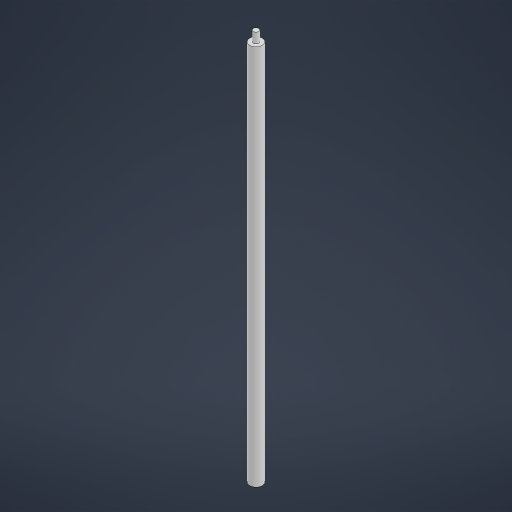
# Autodesk Inventor part: BaseSpacer_M3
Saved by Autodesk Inventor 2024.2 (Build 282272000, 272)
## iProperties
Created: 2023-12-28
Part Number: BaseSpacer_M3
Material: 一般
Document SubType Name: Modeling
Designer: Hanaoka
Density: 1 g/cm^3
Appearance: 既定
Author: Hanaoka
Autodesk Inventor part; units mm, degrees
ref_plane "YZ Plane" through (0, 0, 0) normal (1, 0, 0) x (0, 1, 0)
ref_plane "XZ Plane" through (0, 0, 0) normal (0, 1, 0) x (-1, 0, 0)
ref_plane "XY Plane" through (0, 0, 0) normal (0, 0, 1) x (1, 0, 0)
sketch "スケッチ2" plane through (0, 0, 0) normal (0, 0, 1) x (1, 0, 0)
  line L0 (0, 0) -> (2.5, 0)
  line L1 (2.5, 0) -> (2.5, 150)
  line L2 (2.5, 150) -> (0, 150)
  line L3 (0, 150) -> (0, 0)
  line L4 (1.1, 0) -> (1.1, 6)
  line L5 (1.1, 6) -> (0, 6)
  line L6 (1.1, 150) -> (1.1, 154)
  line L7 (1.1, 154) -> (0, 154)
  line L8 (0, 154) -> (0, 150)
  dimension "d4" = 2.5
  dimension "d5" = 150
  dimension "d6" = 1.1
  dimension "d7" = 6
  dimension "d8" = 1.1
  dimension "d9" = 4
  constraints: 18 end point, 5 perpendicular, 4 point on line, 3 vertical, 1 horizontal
  measures "d4" distance of L0.start L0.end
  measures "d5" distance of L0.end L1.end
  measures "d6" distance of L4.end L5.end
  measures "d7" distance of L4.start L4.end
  measures "d8" distance of L6.end L7.end
  measures "d9" distance of L6.start L6.end
revolve "回転1" add sketch "スケッチ2" angle 360 about axis through (0, 150, 0) along (0, -1, 0) contours L4 L5 L3 L2 L1 L0 | L8 L7 L6 L2
